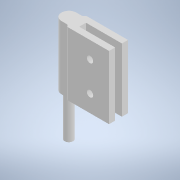
# Autodesk Inventor part: joint male
Saved by Autodesk Inventor 2020 (Build 240168000, 168)
## iProperties
Created: 2020-05-02
Part Number: joint male
Material: Generic
Document SubType Name: Modeling
Designer: galaxy
Density: 1 g/cm^3
Appearance: Default
Author: galaxy
Autodesk Inventor part; units mm, degrees
ref_plane "YZ Plane" through (0, 0, 0) normal (1, 0, 0) x (0, 1, 0)
ref_plane "XZ Plane" through (0, 0, 0) normal (0, 1, 0) x (-1, 0, 0)
ref_plane "XY Plane" through (0, 0, 0) normal (0, 0, 1) x (1, 0, 0)
sketch "Sketch1" plane through (0, 0, 0) normal (0, 1, 0) x (-1, 0, 0)
  line L0 (9.2679, -4.5) -> (-10, -4.5)
  line L1 (-10, 4.5) -> (9.2679, 4.5)
  line L2 (10, -4.5) -> (-10, 4.5) construction
  line L3 (-10, -4.5) -> (10, 4.5) construction
  arc A0 (13.5, -3.5) -> (13.5, 3.5) centre (13.5, 0) ccw
  line L4 (13.5, -3.5) -> (11, -3.5)
  line L5 (13.5, 3.5) -> (11, 3.5)
  line L6 (-10, -1.6) -> (7, -1.6)
  line L7 (7, -1.6) -> (7, 1.6)
  line L8 (7, 1.6) -> (-10, 1.6)
  line L9 (-10, -4.5) -> (-10, -1.6)
  line L10 (-10, 1.6) -> (-10, 4.5)
  line L11 (10, 4.5) -> (10, 4.5)
  line L12 (10, -4.5) -> (10, -4.5)
  arc A1 (11, -3.5) -> (10.134, -4) centre (11, -4.5) ccw
  arc A2 (10.134, 4) -> (11, 3.5) centre (11, 4.5) ccw
  arc A3 (9.2679, -4.5) -> (10.134, -4) centre (9.2679, -3.5) ccw
  arc A4 (10.134, 4) -> (9.2679, 4.5) centre (9.2679, 3.5) ccw
  point P0 (0, 0)
  dimension "d24" = 20
  dimension "d25" = 9
  dimension "d26" = 7
  dimension "d27" = 2.9
  dimension "d28" = 2.9
  dimension "d30" = 1
  constraints: 26 end point, 12 point on circle, 11 tangent, 8 parallel, 6 perpendicular, 5 centre point, 3 equal radius, 2 horizontal, 2 midpoint, 2 point on line
  measures "d24" distance of L1.start L3.end
  measures "d25" distance of L0.end L1.start
  measures "d26" diameter of A0
  measures "d27" distance between parallel lines of L0 L6
  measures "d28" distance between parallel lines of L1 L8
  measures "d30" radius of A1
extrude "Extrusion4" add sketch "Sketch1" along normal blind 30
sketch "Sketch4" plane through (0, 0, 0) normal (0, -1, 0) x (1, 0, 0)
  arc A0 (-13.5, 3.5) -> (-13.5, -3.5) centre (-13.5, 0) ccw projected
  circle A1 centre (-13.5, 0) radius 2
  point P0 (0, 0)
  dimension "d33" = 4
  constraints: 1 centre point, 1 coincident
  measures "d33" diameter of A1
extrude "Extrusion5" add sketch "Sketch4" along normal blind 20
sketch "Sketch5" plane through (-9.2679, 0, 4.5) normal (0, 0, 1) x (1, 0, 0)
  circle A0 centre (10.2679, 22) radius 1.5
  circle A1 centre (10.2679, 8) radius 1.5
  line L0 (19.2679, 0) -> (19.2679, 30) projected
  line L1 (0, 30) -> (19.2679, 30) projected
  line L2 (0, 0) -> (19.2679, 0) projected
  point P0 (9.2679, 0)
  dimension "d36" = 3
  dimension "d37" = 3
  dimension "d38" = 9
  dimension "d39" = 9
  dimension "d40" = 8
  dimension "d41" = 8
  constraints: 2 centre point
  measures "d36" diameter of A0
  measures "d37" diameter of A1
  measures "d38" distance from line of L0 A0.centre
  measures "d39" distance from line of L0 A1.centre
  measures "d40" distance from line of L1 A0.centre
  measures "d41" distance from line of L2 A1.centre
extrude "Extrusion6" cut sketch "Sketch5" against normal blind 20
body "Solid2"
